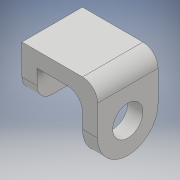
# Autodesk Inventor part: Ex3
Saved by Autodesk Inventor 2018 (Build 220112000, 112)
## iProperties
Created: 2020-11-11
Part Number: Ex3
Material: Generic
Document SubType Name: Modeling
Designer: Neo Yang
Density: 1 g/cm^3
Appearance: Default
Author: Neo Yang
Autodesk Inventor part; units mm, degrees
ref_plane "YZ Plane" through (0, 0, 0) normal (1, 0, 0) x (0, 1, 0)
ref_plane "XZ Plane" through (0, 0, 0) normal (0, 1, 0) x (-1, 0, 0)
ref_plane "XY Plane" through (0, 0, 0) normal (0, 0, 1) x (1, 0, 0)
sketch "Sketch1" plane through (0, 0, 0) normal (0, 1, 0) x (-1, 0, 0)
  line L0 (0, 0) -> (10, 0)
  arc A0 (10, 0) -> (0, -10) centre (10, -10) ccw
  line L1 (0, -20) -> (10, -20)
  arc A1 (20, -10) -> (10, -20) centre (20, -20) ccw
  line L2 (0, -10) -> (0, -20)
  line L3 (10, 0) -> (50.06, 0)
  line L4 (50.06, 0) -> (50.06, -30)
  line L5 (50.06, -30) -> (40.06, -30)
  line L6 (40.06, -30) -> (40.06, -10)
  line L7 (40.06, -10) -> (20, -10)
  dimension "d2" = 20
  dimension "d3" = 50.06
  dimension "d4" = 30
  dimension "d5" = 10
  dimension "d6" = 20
  constraints: 16 end point, 4 horizontal, 4 point on circle, 3 vertical, 2 centre point, 1 tangent
  measures "d2" diameter of A1
  measures "d3" distance of L3.end L0.start
  measures "d4" distance of L3.end L4.end
  measures "d5" distance of L4.end L5.end
  measures "d6" distance of L5.end L6.end
extrude "Extrusion1" add sketch "Sketch1" along normal blind 40
fillet "Fillet1" radius 10 2 edges at (-45.06, 40, -30) (-45.06, 0, -30)
sketch "Sketch3" plane through (0, 0, -10) normal (1, 0, 0) x (0, 0, -1)
  line L0 (10, 0) -> (20, 0)
  line L1 (0, 40) -> (10, 40) projected
  line L2 (20, 40) -> (10, 40)
  circle A0 centre (20, 20) radius 10
  line L3 (10, 0) -> (10, 40) projected
  arc A1 (20, 0) -> (20, 40) centre (20, 20) ccw
  point P0 (-10, 0)
  dimension "d14" = 10
  constraints: 4 end point, 2 centre point, 2 point on circle, 1 coincident, 1 horizontal, 1 tangent
  measures "d14" distance of L0.end L0.start
extrude "Extrusion3" add sketch "Sketch3" against normal blind 10
body "Solid1"
